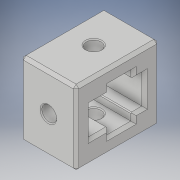
# Autodesk Inventor part: support
Saved by Autodesk Inventor 2019 (Build 230136000, 136)
## iProperties
Created: 2018-05-12
Part Number: support
Material: Générique
Document SubType Name: Modeling
Designer: Theo
Density: 1 g/cm^3
Appearance: Par défaut
Author: Theo
Autodesk Inventor part; units mm, degrees
ref_plane "YZ Plane" through (0, 0, 0) normal (1, 0, 0) x (0, 1, 0)
ref_plane "XZ Plane" through (0, 0, 0) normal (0, 1, 0) x (-1, 0, 0)
ref_plane "XY Plane" through (0, 0, 0) normal (0, 0, 1) x (1, 0, 0)
sketch "Esquisse1" plane through (0, 0, 0) normal (1, 0, 0) x (0, 1, 0)
  line L0 (20, 22.5) -> (-20, 22.5)
  line L1 (-20, 22.5) -> (-20, -22.5)
  line L2 (-20, -22.5) -> (20, -22.5)
  line L3 (20, -22.5) -> (20, 22.5)
  line L4 (8, 14.5) -> (-8, 14.5)
  line L5 (-8, 14.5) -> (-8, 4.5)
  line L6 (-8, 4.5) -> (-12, 4.5)
  line L7 (-12, 4.5) -> (-12, -8.5)
  line L8 (-12, -8.5) -> (-8, -8.5)
  line L9 (8, -14.5) -> (-8, -14.5)
  line L10 (-8, -8.5) -> (-8, -14.5)
  line L11 (8, 14.5) -> (8, 4.5)
  line L12 (8, 4.5) -> (12, 4.5)
  line L13 (12, 4.5) -> (12, -8.5)
  line L14 (12, -8.5) -> (8, -8.5)
  line L15 (8, -14.5) -> (8, -8.5)
  point P0 (0, 0)
  point P1 (-20, 0)
  point P2 (0, -22.5)
  dimension "d8" = 8
  dimension "d9" = 8
  dimension "d15" = 10
  dimension "d33" = 8
  dimension "d35" = 13
  dimension "d36" = 6
  dimension "d38" = 8
  dimension "d40" = 24
  dimension "d41" = 16
  dimension "d42" = 4
  constraints: 32 end point, 7 horizontal, 6 vertical, 5 collinear, 2 midpoint, 2 parallel, 1 horizontal alignment, 1 perpendicular, 1 vertical alignment
  measures "d8" distance between parallel lines of L4 L0
  measures "d9" distance between parallel lines of L7 L1
  measures "d15" distance of L5.end L4.end
  measures "d33" distance between parallel lines of L2 L9
  measures "d35" distance between parallel lines of L8 L6
  measures "d36" distance of L8.end L9.end
  measures "d38" distance between parallel lines of L3 L13
  measures "d40" distance between parallel lines of L7 L13
  measures "d41" distance between parallel lines of L11 L5
  measures "d42" distance of L5.end L6.end
extrude "Extrusion1" add sketch "Esquisse1" along normal blind 30
sketch "Esquisse2" plane through (0, -20, 22.5) normal (0, 0, 1) x (1, 0, 0)
  line L0 (30, 0) -> (0, 0) projected
  line L1 (0, 0) -> (0, 40) projected
  line L2 (0, 40) -> (30, 40) projected
  line L3 (30, 40) -> (30, 0) projected
  circle A0 centre (15, 20) radius 4
  line L4 (0, 28) -> (0, 12) projected
  line L5 (0, 28) -> (30, 28) projected
  line L6 (30, 12) -> (30, 28) projected
  line L7 (0, 12) -> (30, 12) projected
  line L8 (0, 40) -> (30, 40) projected
  point P0 (0, 20)
  point P1 (0, 20)
  point P2 (15, 40)
  point P3 (15, 40)
  point P4 (0, 20)
  dimension "d19" = 8
  constraints: 4 midpoint, 1 centre point, 1 horizontal alignment, 1 vertical alignment
  measures "d19" diameter of A0
extrude "Extrusion2" cut sketch "Esquisse2" against normal up to surface (8 mm away) contours A0
sketch "Esquisse4" plane through (0, -20, -22.5) normal (0, -1, 0) x (1, 0, 0)
  line L0 (0, 27) -> (0, 14) projected
  line L1 (0, 27) -> (30, 27) projected
  line L2 (30, 14) -> (30, 27) projected
  line L3 (0, 14) -> (30, 14) projected
  circle A0 centre (15, 20.5) radius 4
  point P0 (0, 22.5)
  point P1 (30, 20.5)
  point P2 (15, 27)
  dimension "d24" = 8
  constraints: 2 midpoint, 1 centre point, 1 horizontal alignment, 1 vertical alignment
  measures "d24" diameter of A0
extrude "Extrusion3" cut sketch "Esquisse4" against normal up to surface (40 mm away) contours A0
chamfer "Chanfrein1" distance 1.5 angle 45 36 edges at (15, 20, -22.5) (15, -20, -22.5) (15, -20, 22.5) (15, 20, 22.5) (30, 20, 0) (30, 0, -22.5) (0, 0, -22.5) (0, 20, 0) (30, 0, 22.5) (0, 0, 22.5) (0, -20, 0) (30, -20, 0) (30, -12, -2) (30, -10, 4.5) (30, -8, 9.5) (30, 0, 14.5) (0, -12, -2) (0, -8, 9.5) (0, 0, 14.5) (0, -10, 4.5) (0, -10, -8.5) (0, -8, -11.5) (0, 0, -14.5) (30, -10, -8.5) (30, -8, -11.5) (30, 0, -14.5) (30, 8, 9.5) (30, 12, -2) (30, 10, 4.5) (30, 10, -8.5) (30, 8, -11.5) (0, 8, -11.5) (0, 10, -8.5) (0, 12, -2) (0, 10, 4.5) (0, 8, 9.5)
chamfer "Chanfrein2" distance 0.5 angle 45 10 edges at (11, 0, 14.5) (11, 0, 22.5) (11, -12, -2) (11, 20, -2) (11, -20, -2) (15, -8, 4.5) (15, -8, -8.5) (11, 12, -2) (15, 8, -8.5) (15, 8, 4.5)
equation "\"d8\" = d6"
equation "\"d9\" = d6"
equation "\"d6\" = 8"
